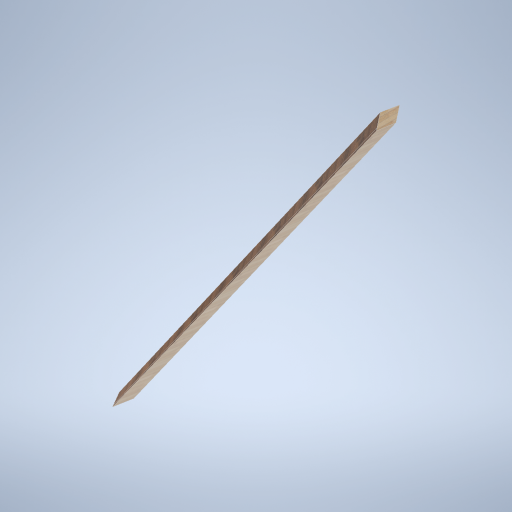
# Autodesk Inventor part: side_curve_panel_01
Saved by Autodesk Inventor 2024.2 (Build 282272000, 272)
## iProperties
Created: 2024-05-24
Part Number: side_curve_panel_01
Material: Wood (Maple)
Document SubType Name: Modeling
Designer: LOSTER_1
Density: 0.67 g/cm^3
Appearance: Natural Maple - Glossy Dark Tint
Author: LOSTER_1
Autodesk Inventor part; units mm, degrees
ref_plane "XZ Plane" through (0, 0, 0) normal (0, 1, 0) x (-1, 0, 0)
ref_plane "XY Plane" through (0, 0, 0) normal (0, 0, 1) x (1, 0, 0)
sketch "Sketch13" plane through (0, 0, 0) normal (1, 0, 0) x (0, 1, 0)
  arc A0 (55855.2929, -6406.0695) -> (55878.8004, -6254.966) centre (-62706.6016, 12116.2733) ccw
  ellipse E0 centre (61807.5968, 1929.0762) end of major axis (51807.5968, 1929.344) minor radius 9999.9998 (55917.1825, -6151.952) -> (56015.6856, -6222.8415) ccw
  ellipse E1 centre (19397.9187, -2349.5656) end of major axis (39154.6168, -37129.9174) minor radius 39999.9568 (59006.8331, -7929.1471) -> (59041.0479, -7680.6172) ccw construction
  arc A1 (55855.2929, -6406.0695) -> (55896.9861, -6137.1918) centre (-62706.6016, 12116.2733) ccw
  arc A2 (59006.8331, -7929.1471) -> (59041.0479, -7680.6172) centre (19397.8959, -2349.6046) ccw
  line L0 (59041.0479, -7680.6172) -> (59220.0192, -7728.5691)
  arc A3 (59178.0471, -7975.0206) -> (59220.0192, -7728.5691) centre (44232.9887, -5302.9896) ccw
  line L1 (59178.0471, -7975.0206) -> (59006.8331, -7929.1471)
  arc A4 (55896.9861, -6137.1918) -> (55917.1825, -6151.952) centre (61807.5968, 1929.0762) ccw
  arc A5 (59041.0527, -7680.6185) -> (59219.7435, -7730.2723) centre (61807.5968, 1929.0762) ccw
  arc A6 (55968.67, -6468.3808) -> (56015.6856, -6222.8415) centre (48135.8799, -4841.298) ccw
  line L2 (55968.67, -6468.3808) -> (55855.2929, -6406.0695)
  point P0 (0, 0)
  point P1 (-3.2447, -8.5693)
  dimension "d19" = 250
  dimension "d20" = 250
  dimension "d21" = 8000
  constraints: 15 point on circle, 7 centre point, 6 end point, 1 coincident, 1 point on line, 9 other
  measures "d19" distance of L0.end L1.start
  measures "d20" distance of A6.end L2.start
  measures "d21" radius of A6
ref_plane "Work Plane9" through (1791, 0, 0) normal (1, 0, 0) x (0, 1, 0)
ref_plane "Work Plane8" through (0, 0, 0) normal (1, 0, 0) x (0, 1, 0)
sketch "Sketch14" plane through (1791, 0, 0) normal (1, 0, 0) x (0, 1, 0)
  ellipse E0 centre (19397.9187, -2349.5656) end of major axis (39154.6168, -37129.9174) minor radius 39999.9568 (59006.8331, -7929.1471) -> (59041.0479, -7680.6172) ccw construction
  line L0 (59178.0471, -7975.0206) -> (59006.8331, -7929.1471) projected
  arc A0 (59006.8331, -7929.1471) -> (59041.0527, -7680.6185) centre (19397.9942, -2348.8351) ccw
  line L1 (59006.8331, -7929.1471) -> (59178.0471, -7975.0206)
  arc A1 (59178.0471, -7975.0206) -> (59219.7435, -7730.2723) centre (44232.9887, -5302.9896) ccw
  line L2 (59041.0527, -7680.6185) -> (59219.7435, -7730.2723)
  point P0 (0, 0)
  dimension "d24" = 40000
  constraints: 4 end point, 4 point on circle, 2 centre point, 1 collinear, 1 point on line, 1 other
  measures "d24" radius of A0
sketch "Sketch15" plane through (0, 0, 0) normal (1, 0, 0) x (0, 1, 0)
  arc A0 (55855.2929, -6406.0695) -> (55896.9861, -6137.1918) centre (-62706.6016, 12116.2733) ccw projected
  line L0 (55968.67, -6468.3808) -> (55855.2929, -6406.0695) projected
  arc A1 (55968.67, -6468.3808) -> (56015.6856, -6222.8415) centre (48135.8799, -4841.298) ccw projected
  ellipse E0 centre (61807.5968, 1929.0762) end of major axis (51807.5968, 1929.344) minor radius 9999.9998 (55917.1825, -6151.952) -> (56015.6856, -6222.8415) ccw projected
  arc A2 (55896.9861, -6137.1918) -> (55917.1825, -6151.952) centre (61807.5968, 1929.0762) ccw projected
  constraints: 1 other
loft "Loft4" add profiles "Sketch14", "Sketch15"
body "Solid4"
